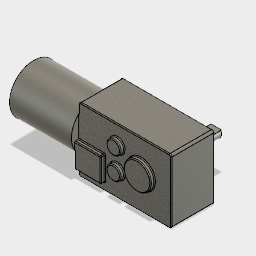
Gear Motor ZWL-FP69i v8 (Autodesk Fusion 360 design; units mm, degrees)
Autodesk Fusion 360 part; units mm, degrees
sketch "Sketch1" plane through (0, 0, 0) normal (0, 1, 0) x (1, 0, 0)
  line L0 (0, 0) -> (46, 0)
  line L1 (46, 0) -> (46, 21.4)
  line L2 (46, 21.4) -> (0, 21.4)
  line L3 (0, 21.4) -> (0, 0)
  line L4 (-30.8, 20.52) -> (0, 20.52)
  line L5 (0, 20.52) -> (0, -3.58)
  line L6 (0, -3.58) -> (-30.8, -3.58)
  line L7 (-30.8, -3.58) -> (-30.8, 20.52)
  line L8 (0, 21.4) -> (0, 20.52)
  dimension "d1" = 21.4
  dimension "d2" = 46
  dimension "d3" = 30.8
  dimension "d4" = 24.1
  dimension "d5" = 0.88
  measures "d1" distance of L0.start L2.end
  measures "d2" distance of L0.start L0.end
  measures "d3" distance of L4.start L4.end
  measures "d4" distance of L4.start L6.end
  measures "d5" distance of L2.end L4.end
extrude "Extrude1" add sketch "Sketch1" along normal blind 32 contours L0 L1 L2 L3 L5 L8
sketch "Sketch2" plane through (0, 0, 0) normal (-1, 0, 0) x (0, 0, 1)
  line L0 (-21.4, 0) -> (0, 0)
  line L1 (0, 0) -> (0, 32)
  line L2 (0, 32) -> (-21.4, 32)
  line L3 (-21.4, 32) -> (-21.4, 0)
  line L4 (3.58, 0) -> (-20.52, 0)
  line L5 (3.58, 0) -> (-20.52, 0)
  line L6 (-20.52, 0) -> (-20.52, 18.1033) construction
  line L7 (-20.52, 18.1033) -> (3.58, 18.1033) construction
  line L8 (3.58, 18.1033) -> (3.58, 0) construction
  circle A0 centre (-8.47, 18.1033) radius 12.05
  line L9 (-9.0363, 32) -> (-9.0363, 30.14) construction
  point P0 (-20.52, 0)
  point P1 (3.58, 0)
  dimension "d8" = 1.86
  measures "d8" distance of L9.start L9.end
extrude "Extrude2" add sketch "Sketch2" along normal up to surface (30.8 mm away) contours L1 A0 | L1 A0
sketch "Sketch3" plane through (0, 0, -21.4) normal (0, 0, -1) x (-1, 0, 0)
  line L0 (-46, 0) -> (0, 0)
  line L1 (0, 0) -> (0, 32)
  line L2 (0, 32) -> (-46, 32)
  line L3 (-46, 32) -> (-46, 0)
  circle A0 centre (-40, 25.5) radius 3.95
  circle A1 centre (-40, 25.5) radius 1.5
  line L4 (-40, 25.5) -> (-7, 25.5) construction
  line L5 (-7, 25.5) -> (-7, 7.5) construction
  line L6 (-7, 7.5) -> (-40, 7.5) construction
  line L7 (-40, 7.5) -> (-40, 25.5) construction
  circle A2 centre (-7, 25.5) radius 1.5
  circle A3 centre (-7, 25.5) radius 3.95
  circle A4 centre (-40, 7.5) radius 1.5
  circle A5 centre (-40, 7.5) radius 3.95
  circle A6 centre (-7, 7.5) radius 1.5
  circle A7 centre (-7, 7.5) radius 3.95
  circle A8 centre (-31, 16.5) radius 6.75
  circle A9 centre (-31, 16.5) radius 3
  circle A10 centre (-19.2, 22.8) radius 3.5
  circle A11 centre (-19.2, 11.8) radius 3.5
  line L8 (-19.2, 11.8) -> (-19.2, 22.8) construction
  dimension "d11" = 7.9
  dimension "d12" = 3
  dimension "d13" = 33
  dimension "d14" = 18
  dimension "d16" = 6
  dimension "d17" = 6.5
  dimension "d18" = 9
  dimension "d19" = 9
  dimension "d20" = 13.5
  dimension "d21" = 6
  dimension "d22" = 7
  dimension "d23" = 7
  dimension "d24" = 20.8
  dimension "d25" = 2.7
  dimension "d26" = 11
  measures "d11" diameter of A0
  measures "d12" diameter of A1
  measures "d13" distance of A0.centre L4.end
  measures "d14" distance of A0.centre L6.end
  measures "d16" distance of L3 A0.centre
  measures "d17" distance of L2 A0.centre
  measures "d18" distance of L7 A8.centre
  measures "d19" distance of L4 A8.centre
  measures "d20" diameter of A8
  measures "d21" diameter of A9
  measures "d22" diameter of A10
  measures "d23" diameter of A11
  measures "d24" distance of L7 L8
  measures "d25" distance of L4 A10.centre
  measures "d26" distance of A11.centre A10.centre
extrude "Extrude3" add sketch "Sketch3" along normal blind 2 contours A0 | A3 | A5 | A7 | A8 | A10 | A11
extrude "Extrude4" add 1 faces at (31.7906, 15.5676, -21.4) along direction (0, 0, -1) blind 16
extrude "Extrude5" cut 4 faces at (7.3832, 8.062, -21.4) (7.3384, 25.2183, -21.4) (39.6168, 24.938, -21.4) (40.0399, 7.0346, -21.4) along direction (0, 0, 1) blind 7
sketch "Sketch4" plane through (0, 0, 0) normal (0, 0, 1) x (1, 0, 0)
  line L0 (0, 0) -> (46, 0)
  line L1 (46, 0) -> (46, 32)
  line L2 (46, 32) -> (0, 32)
  line L3 (0, 32) -> (0, 26.6743)
  line L4 (0, 26.6743) -> (0, 9.5323)
  line L5 (0, 9.5323) -> (0, 0)
  line L6 (46, 0) -> (0, 0)
  line L7 (0, 0) -> (0, 32)
  line L8 (0, 32) -> (46, 32)
  line L9 (46, 32) -> (46, 0)
  circle A0 centre (19.2, 22.8) radius 3.5
  circle A1 centre (19.2, 11.8) radius 3.5
  circle A2 centre (31, 16.5) radius 6.75
  line L10 (0, 15.88) -> (13, 15.88)
  line L11 (13, 15.88) -> (13, 3.88)
  line L12 (13, 3.88) -> (0, 3.88)
  line L13 (0, 3.88) -> (0, 15.88)
  dimension "d33" = 13
  dimension "d34" = 12
  dimension "d35" = 3.88
  measures "d33" distance of L10.start L10.end
  measures "d34" distance of L10.start L12.end
  measures "d35" distance of L0 L11.end
extrude "Extrude6" add sketch "Sketch4" along normal blind 2 contours L4 L5 L7 L10 L11 L12 L13 | A0 | A1 | A2
fillet "Fillet1" radius 1 4 edges at (0, 0, -10.7) (46, 0, -10.7) (0, 32, -10.7) (46, 32, -10.7)
fillet "Fillet2" radius 0.4 47 edges at (23, 32, -21.4) (0.2929, 31.7071, -21.4) (0, 16, -21.4) (0.2929, 0.2929, -21.4) (23, 0, -21.4) (45.7071, 0.2929, -21.4) (46, 16, -21.4) (45.7071, 31.7071, -21.4) (43.6827, 26.9284, -21.4) (43.6827, 24.0716, -23.4) (43.6827, 8.9284, -21.4) (43.6827, 6.0716, -23.4) (22.4631, 10.5343, -23.4) (22.4631, 13.0657, -21.4) (10.6827, 8.9284, -21.4) (10.6827, 6.0716, -23.4) (10.6827, 24.0716, -23.4) (10.6827, 26.9284, -21.4) (22.4631, 21.5343, -23.4) (37.2932, 14.0591, -23.4) (37.2932, 18.9409, -21.4) (22.4631, 24.0657, -21.4) (0, 28.8371, 0) (0.2929, 31.7071, 0) (23, 32, 0) (45.7071, 31.7071, 0) (46, 16, 0) (45.7071, 0.2929, 0) (23, 0, 0) (0.2929, 0.2929, 0) (0, 2.44, 0) (24.7068, 14.0591, 2) (24.7068, 18.9409, 0) (15.9369, 24.0657, 0) (15.9369, 21.5343, 2) (15.9369, 13.0657, 0) (15.9369, 10.5343, 2) (6.5, 15.88, 0) (6.5, 15.88, 2) (13, 9.88, 0) (13, 15.88, 1) (13, 3.88, 1) (13, 9.88, 2) (6.5, 3.88, 0) (0, 3.88, 1) (0, 8.0091, 2) (6.5, 3.88, 2)
fillet "Fillet3" radius 0.4 1 edges at (33.797, 15.4152, -37.4)
sketch "Sketch5" plane through (0, 0, -37.4) normal (0, 0, -1) x (-1, 0, 0)
  circle A0 centre (-31, 16.5) radius 2.6
  circle A1 centre (-31, 16.5) radius 3
  circle A2 centre (-31, 16.5) radius 3
  line L0 (-33.6317, 17.9401) -> (-28.3683, 17.9401)
  line L1 (-31.0251, 17.9401) -> (-31.0251, 13.5001) construction
  dimension "d41" = 4.44
  measures "d41" distance of L1.start L1.end
extrude "Extrude7" cut sketch "Sketch5" against normal blind 11 contours A0 L0 | A0 A1 A2 L0 picked at (-31.3547, 18.2508) picked at (-31, 19.3616)
